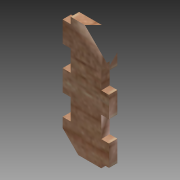
# Autodesk Inventor part: tussenplaatje
Saved by Autodesk Inventor 2015 (Build 190159000, 159)
## iProperties
Created: 2016-01-23
Part Number: tussenplaatje
Material: Generic
Document SubType Name: Modeling
Designer: david
Density: 1 g/cm^3
Appearance: Birch - Natural Polished
Author: david
Autodesk Inventor part; units mm, degrees
ref_plane "YZ Plane" through (0, 0, 0) normal (1, 0, 0) x (0, 1, 0)
ref_plane "XZ Plane" through (0, 0, 0) normal (0, 1, 0) x (-1, 0, 0)
ref_plane "XY Plane" through (0, 0, 0) normal (0, 0, 1) x (1, 0, 0)
sketch "Sketch1" plane through (0, 0, 0) normal (0, 1, 0) x (-1, 0, 0)
  line L0 (-7.25, 27.5) -> (7.25, 27.5)
  line L1 (7.25, 27.5) -> (7.25, -27.5)
  line L2 (7.25, -27.5) -> (-7.25, -27.5)
  line L3 (-7.25, -27.5) -> (-7.25, 27.5)
  line L4 (-7.25, 27.5) -> (7.25, -27.5) construction
  line L5 (7.25, 27.5) -> (-7.25, -27.5) construction
  point P0 (0, 0)
  dimension "d0" = 14.5
  dimension "d1" = 55
  constraints: 12 end point, 2 midpoint, 2 parallel, 1 horizontal, 1 perpendicular
  measures "d0" distance of L1.end L2.end
  measures "d1" distance of L0.end L1.end
extrude "Extrusion1" add sketch "Sketch1" along normal blind 4
sketch "Sketch2" plane through (0, 4, 0) normal (0, 1, 0) x (1, 0, 0)
  line L0 (0, -21.4425) -> (0, 24.9563)
  line L1 (6.9273, -24.5) -> (10.9273, -24.5)
  line L2 (10.9273, -24.5) -> (10.9273, -14.5)
  line L3 (10.9273, -14.5) -> (6.9273, -14.5)
  line L4 (6.9273, -14.5) -> (6.9273, -24.5)
  line L5 (7.25, -27.5) -> (-7.25, -27.5) projected
  point P0 (0, 0)
  dimension "d10" = 4
  dimension "d11" = 10
  dimension "d12" = 3
  constraints: 10 end point, 2 parallel, 1 horizontal, 1 perpendicular, 1 vertical
  measures "d10" distance of L3.end L2.end
  measures "d11" distance of L2.end L1.end
  measures "d12" distance between parallel lines of L5 L1
extrude "Extrusion2" add sketch "Sketch2" against normal blind 4
pattern_linear "Rectangular Pattern1" count 3 spacing 20 along (0, 0, -1) count 2 spacing 18 along (-1, 0, 0) of "Extrusion2"
body "Solid1"
